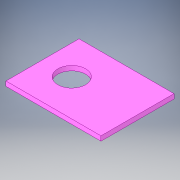
# Autodesk Inventor part: Hombro_sostenedorcojin
Saved by Autodesk Inventor 2019 (Build 230136000, 136)
## iProperties
Created: 2020-02-08
Part Number: Hombro_sostenedorcojin
Material: Generic
Document SubType Name: Modeling
Designer: Omar
Density: 1 g/cm^3
Appearance: Default
Author: Omar
Autodesk Inventor part; units mm, degrees
ref_plane "YZ Plane" through (0, 0, 0) normal (1, 0, 0) x (0, 1, 0)
ref_plane "XZ Plane" through (0, 0, 0) normal (0, 1, 0) x (-1, 0, 0)
ref_plane "XY Plane" through (0, 0, 0) normal (0, 0, 1) x (1, 0, 0)
sketch "Sketch1" plane through (0, 0, 0) normal (0, 1, 0) x (-1, 0, 0)
  line L0 (20, 25) -> (-45, 25)
  line L1 (-45, 25) -> (-45, -25)
  line L2 (-45, -25) -> (20, -25)
  line L3 (20, -25) -> (20, 25)
  circle A0 centre (0, 0) radius 9.5
  dimension "d11" = 50
  dimension "d12" = 65
  dimension "d13" = 25
  dimension "d20" = 20
  dimension "d21" = 19
  constraints: 8 end point, 3 coincident, 2 parallel, 1 centre point, 1 horizontal, 1 perpendicular
  measures "d11" distance of L0.end L1.end
  measures "d12" distance of L0.start L0.end
  measures "d13" distance from line of L0 point (0, 0)
  measures "d20" distance from line of L3 point (0, 0)
  measures "d21" diameter of A0
extrude "Extrusion1" add sketch "Sketch1" along normal blind 3.18
body "Solid1"
